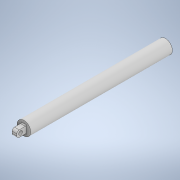
# Autodesk Inventor part: linear_actuator_LH
Saved by Autodesk Inventor 2021 (Build 250183000, 183)
## iProperties
Created: 2021-06-25
Part Number: linear_actuator_LH
Material: Generic
Document SubType Name: Modeling
Density: 1 g/cm^3
Appearance: Default
Mass: 243.882 g
Surface Area: 328.805 cm^2
Volume: 243.882 cm^3
Autodesk Inventor part; units mm, degrees
ref_plane "YZ Plane" through (0, 0, 0) normal (1, 0, 0) x (0, 1, 0)
ref_plane "XZ Plane" through (0, 0, 0) normal (0, 1, 0) x (-1, 0, 0)
ref_plane "XY Plane" through (0, 0, 0) normal (0, 0, 1) x (1, 0, 0)
sketch "Sketch1" plane through (0, 0, 0) normal (0, 0, 1) x (1, 0, 0)
  circle A0 centre (0, 0) radius 14.5
  dimension "d6" = 29
  constraints: 1 centre point
  measures "d6" diameter of A0
extrude "Extrusion3" add sketch "Sketch1" along normal blind 300
sketch "Sketch3" plane through (0, 0, 0) normal (1, 0, 0) x (0, 1, 0)
  line L0 (-7, 295.5461) -> (7, 295.5461)
  line L1 (7, 295.5461) -> (7, 320)
  line L2 (7, 320) -> (-7, 320)
  line L3 (-7, 320) -> (-7, 295.5461)
  line L4 (0, 384) -> (0, -64) projected
  line L5 (14.5, 300) -> (-14.5, 300) projected
  point P0 (0, 0)
  point P1 (7, 300)
  point P2 (-7, 300)
  dimension "d9" = 7
  dimension "d10" = 7
  dimension "d11" = 20
  constraints: 8 end point, 2 parallel, 1 horizontal, 1 perpendicular
  measures "d9" distance between parallel lines of L4 L3
  measures "d10" distance between parallel lines of L4 L1
  measures "d11" distance between parallel lines of L5 L2
extrude "Extrusion4" add sketch "Sketch3" along normal mid plane 10 contours L3 L2 L4 L5 | L4 L2 L1 L5
fillet "Fillet1" radius 2 2 edges at (0, -7, 300) (0, 7, 300)
fillet "Fillet2" radius 5 2 edges at (0, -7, 320) (0, 7, 320)
sketch "Sketch4" plane through (5, 0, 0) normal (1, 0, 0) x (0, 0, -1)
  line L0 (-320, 2) -> (-320, -2) projected
  point P0 (0, 0)
  point P1 (-312, 0)
  dimension "d16" = 8
  measures "d16" distance from line of L0 point (-312, 0)
hole "Hole1" at (5, 0, 312) direction (-1, 0, 0) diameter 8 end through all
equation "\"d10\" = d9"
body "Solid3"
